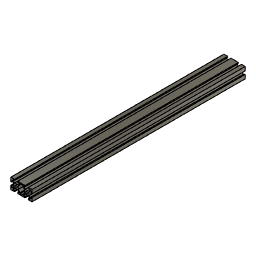
20x40 Extrusion v1 (Autodesk Fusion 360 design; units mm, degrees)
Autodesk Fusion 360 part; units mm, degrees
sketch "Sketch1" plane through (0, 0, 0) normal (0, 1, 0) x (1, 0, 0)
  line L0 (-13, -4) -> (-7, -4)
  line L1 (7, -4) -> (13, -4)
  line L2 (14, -3) -> (14, 3)
  line L3 (13, 4) -> (7, 4)
  line L4 (-7, 4) -> (-13, 4)
  line L5 (-14, 3) -> (-14, -3)
  line L6 (-13, -10) -> (-13, -8)
  line L7 (-7, -10) -> (-7, -8)
  line L8 (7, -10) -> (7, -8)
  line L9 (13, -10) -> (13, -8)
  line L10 (18, -3) -> (20, -3)
  line L11 (18, 3) -> (20, 3)
  line L12 (13, 8) -> (13, 10)
  line L13 (7, 8) -> (7, 10)
  line L14 (-7, 8) -> (-7, 10)
  line L15 (-13, 8) -> (-13, 10)
  line L16 (-18, -3) -> (-20, -3)
  line L17 (-20, 3) -> (-18, 3)
  line L18 (-2.5, -6.3787) -> (-2.5, -8)
  line L19 (2.5, -8) -> (2.5, -6.3787)
  line L20 (2.5, -6.3787) -> (6, -2.8787)
  line L21 (6, -2.8787) -> (6, 2.8787)
  line L22 (6, 2.8787) -> (2.5, 6.3787)
  line L23 (2.5, 6.3787) -> (2.5, 8)
  line L24 (-2.5, 8) -> (-2.5, 6.3787)
  line L25 (-2.5, 6.3787) -> (-6, 2.8787)
  line L26 (-6, 2.8787) -> (-6, -2.8787)
  line L27 (-6, -2.8787) -> (-2.5, -6.3787)
  circle A0 centre (-10, 0) radius 2
  circle A1 centre (10, 0) radius 2
  line L28 (4, -8) -> (4, -7)
  line L29 (4, -7) -> (7, -4)
  line L30 (16, -8) -> (16, -7)
  line L31 (16, -7) -> (13, -4)
  line L32 (18, -6) -> (17, -6)
  line L33 (17, -6) -> (14, -3)
  line L34 (18, 6) -> (17, 6)
  line L35 (17, 6) -> (14, 3)
  line L36 (16, 8) -> (16, 7)
  line L37 (16, 7) -> (13, 4)
  line L38 (7, 4) -> (4, 7)
  line L39 (4, 7) -> (4, 8)
  line L40 (-7, 4) -> (-4, 7)
  line L41 (-4, 7) -> (-4, 8)
  line L42 (-13, 4) -> (-16, 7)
  line L43 (-16, 7) -> (-16, 8)
  line L44 (-18, 6) -> (-17, 6)
  line L45 (-17, 6) -> (-14, 3)
  line L46 (-14, -3) -> (-17, -6)
  line L47 (-17, -6) -> (-18, -6)
  line L48 (-16, -7) -> (-13, -4)
  line L49 (-4, -8) -> (-4, -7)
  line L50 (-4, -7) -> (-7, -4)
  line L51 (-16, -7) -> (-16, -8)
  line L52 (-13, 8) -> (-16, 8)
  line L53 (-13, 10) -> (-20, 10)
  line L54 (16, 8) -> (13, 8)
  line L55 (20, 10) -> (13, 10)
  line L56 (7, 10) -> (-7, 10)
  line L57 (18, -6) -> (18, -3)
  line L58 (18, 3) -> (18, 6)
  line L59 (20, -10) -> (20, -3)
  line L60 (20, 3) -> (20, 10)
  line L61 (13, -8) -> (16, -8)
  line L62 (13, -10) -> (20, -10)
  line L63 (-16, -8) -> (-13, -8)
  line L64 (-20, -10) -> (-13, -10)
  line L65 (-7, -10) -> (7, -10)
  line L66 (-18, 6) -> (-18, 3)
  line L67 (-18, -3) -> (-18, -6)
  line L68 (-20, 10) -> (-20, 3)
  line L69 (-20, -3) -> (-20, -10)
  line L70 (-4, 8) -> (-7, 8)
  line L71 (7, 8) -> (4, 8)
  line L72 (2.5, 8) -> (-2.5, 8)
  line L73 (4, -8) -> (7, -8)
  line L74 (-7, -8) -> (-4, -8)
  line L75 (-2.5, -8) -> (2.5, -8)
  dimension "d4" = 40
  dimension "d5" = 20
  dimension "d7" = 20
  dimension "d8" = 10
  dimension "d9" = 6
  dimension "d10" = 6
  dimension "d11" = 6
  dimension "d12" = 6
  dimension "d13" = 6
  dimension "d14" = 6
  dimension "d15" = 6
  dimension "d16" = 6
  dimension "d17" = 6
  dimension "d18" = 6
  dimension "d19" = 6
  dimension "d20" = 6
  dimension "d21" = 7
  dimension "d22" = 7
  dimension "d23" = 7
  dimension "d24" = 4
  dimension "d25" = 4
  dimension "d26" = 10
  dimension "d27" = 10
  dimension "d28" = 10
  dimension "d29" = 10
  dimension "d30" = 12
  dimension "d32" = 12
  dimension "d33" = 135
  dimension "d34" = 135
  dimension "d35" = 3
  dimension "d36" = 135
  dimension "d37" = 135
  dimension "d38" = 3
  dimension "d39" = 7
  dimension "d41" = 12
  dimension "d42" = 3
  dimension "d43" = 7
  dimension "d44" = 3
  dimension "d45" = 3
  dimension "d46" = 135
  dimension "d47" = 135
  dimension "d48" = 7
  dimension "d49" = 3
  dimension "d50" = 3
  dimension "d52" = 135
  dimension "d53" = 135
  dimension "d54" = 135
  dimension "d55" = 135
  dimension "d56" = 8
  dimension "d57" = 8
  dimension "d58" = 3
  dimension "d59" = 3
  dimension "d60" = 6
  dimension "d61" = 6
  dimension "d62" = 6
  dimension "d63" = 135
  dimension "d64" = 6
  dimension "d65" = 6
  dimension "d66" = 6
  dimension "d67" = 7
  dimension "d68" = 7
  dimension "d69" = 7
  dimension "d70" = 7
  dimension "d71" = 135
  dimension "d72" = 7
  dimension "d73" = 7
  dimension "d74" = 1.5
  dimension "d75" = 1.5
  dimension "d76" = 1.5
  dimension "d77" = 1.5
  dimension "d78" = 1.5
  dimension "d79" = 1.5
  dimension "d80" = 1.5
  dimension "d81" = 1.5
  dimension "d82" = 8
  dimension "d83" = 18
  dimension "d84" = 8
  dimension "d85" = 18
  constraint horizontal L55
  constraint perpendicular L55 L68
  constraint parallel L55 L64
  constraint parallel L59 L68
  constraint perpendicular L0 L57
  constraint parallel L1 L63
  constraint parallel L2 L57
  constraint parallel L3 L54
  constraint parallel L4 L54
  constraint perpendicular L4 L5
  constraint perpendicular L6 L63
  constraint coincident L7.start L64
  constraint coincident L7.end L63
  constraint perpendicular L7 L63
  constraint perpendicular L8 L63
  constraint coincident L9.start L64
  constraint coincident L9.end L63
  constraint perpendicular L9 L63
  constraint perpendicular L10 L59
  constraint coincident L11.start L57
  constraint coincident L11.end L59
  constraint perpendicular L11 L59
  constraint perpendicular L12 L54
  constraint coincident L13.start L54
  constraint coincident L13.end L55
  constraint perpendicular L13 L55
  constraint perpendicular L14 L55
  constraint coincident L15.start L54
  constraint coincident L15.end L55
  constraint perpendicular L15 L54
  constraint coincident L16.start L66
  constraint coincident L16.end L68
  constraint perpendicular L16 L68
  constraint perpendicular L17 L66
  constraint coincident L18.end L63
  constraint perpendicular L18 L63
  constraint coincident L19.start L63
  constraint perpendicular L19 L63
  constraint perpendicular L21 L63
  constraint coincident L23.end L54
  constraint perpendicular L23 L54
  constraint coincident L24.start L54
  constraint perpendicular L24 L54
  constraint perpendicular L26 L54
  constraint coincident L28.start L63
  constraint perpendicular L28 L63
  constraint coincident L30.start L63
  constraint perpendicular L30 L63
  constraint perpendicular L32 L57
  constraint coincident L34.start L57
  constraint perpendicular L34 L57
  constraint perpendicular L36 L54
  constraint perpendicular L3 L39
  constraint coincident L39.end L54
  constraint coincident L41.end L54
  constraint perpendicular L41 L54
  constraint perpendicular L4 L43
  constraint coincident L43.end L54
  constraint perpendicular L44 L66
  constraint coincident L47.end L66
  constraint perpendicular L47 L66
  constraint coincident L49.start L63
  constraint perpendicular L49 L63
  constraint perpendicular L51 L63
  constraint parallel L27 L50
  constraint parallel L20 L29
  constraint parallel L22 L38
  constraint parallel L25 L40
  constraint parallel L54 L55
  constraint parallel L66 L68
  constraint parallel L63 L64
  constraint parallel L57 L59
  constraint collinear L52 L54
  constraint collinear L53 L55
  constraint collinear L54 L71
  constraint collinear L55 L56
  constraint collinear L57 L58
  constraint collinear L59 L60
  constraint collinear L61 L63
  constraint collinear L62 L64
  constraint collinear L63 L74
  constraint collinear L64 L65
  constraint collinear L66 L67
  constraint collinear L68 L69
  constraint collinear L70 L71
  constraint collinear L71 L72
  constraint collinear L73 L74
  constraint collinear L74 L75
  measures "d4" distance of L64.start L59.start
  measures "d5" distance of L53.end L64.start
  measures "d7" distance of origin L59
  measures "d8" distance of origin L55
  measures "d9" distance of L1 L64
  measures "d10" distance of L2 L59
  measures "d11" distance of L3 L55
  measures "d12" distance of L4 L55
  measures "d13" distance of L5 L68
  measures "d14" distance of L0 L64
  measures "d15" distance of L6 L7
  measures "d16" distance of L8 L9
  measures "d17" distance of L10 L11
  measures "d18" distance of L12 L13
  measures "d19" distance of L14 L15
  measures "d20" distance of L16 L17
  measures "d21" distance of L16 L64
  measures "d22" distance of L6 L68
  measures "d23" distance of L9 L59
  measures "d24" diameter of A0
  measures "d25" diameter of A1
  measures "d26" distance of origin A1.centre
  measures "d27" distance of A1.centre L64
  measures "d28" distance of origin A0.centre
  measures "d29" distance of A0.centre L64
  measures "d30" distance of L49 L51
  measures "d32" distance of L28 L30
  measures "d33" angle of L1 L31
  measures "d34" angle of L1 L29
  measures "d35" distance of L6 L51
  measures "d36" angle of L0 L48
  measures "d37" angle of L0 L50
  measures "d38" distance of L8 L28
  measures "d39" distance of L10 L64
  measures "d41" distance of L32 L34
  measures "d42" distance of L10 L32
  measures "d43" distance of L12 L59
  measures "d44" distance of L12 L36
  measures "d45" distance of L13 L39
  measures "d46" angle of L3 L37
  measures "d47" angle of L3 L38
  measures "d48" distance of L15 L68
  measures "d49" distance of L15 L43
  measures "d50" distance of L14 L41
  measures "d52" angle of L4 L42
  measures "d53" angle of L4 L40
  measures "d54" angle of L5 L45
  measures "d55" angle of L5 L46
  measures "d56" distance of L5 L26
  measures "d57" distance of L2 L21
  measures "d58" distance of L16 L47
  measures "d59" distance of L17 L44
  measures "d60" distance of L0.start L0.end
  measures "d61" distance of L1.start L1.end
  measures "d62" distance of L2.start L2.end
  measures "d63" angle of L2 L33
  measures "d64" distance of L3.start L3.end
  measures "d65" distance of L4.start L4.end
  measures "d66" distance of L5.start L5.end
  measures "d67" distance of L5.start L55
  measures "d68" distance of L4.end L68
  measures "d69" distance of L3.start L59
  measures "d70" distance of L2.end L55
  measures "d71" angle of L2 L35
  measures "d72" distance of L1.end L59
  measures "d73" distance of L0.start L68
  measures "d74" distance of L20 L29
  measures "d75" distance of L22 L38
  measures "d76" distance of L25 L40
  measures "d77" distance of L27 L50
  measures "d78" distance of L18 L49
  measures "d79" distance of L19 L28
  measures "d80" distance of L23 L39
  measures "d81" distance of L24 L41
  measures "d82" distance of origin L63
  measures "d83" distance of origin L67
  measures "d84" distance of origin L72
  measures "d85" distance of origin L58
extrude "Extrude1" add sketch "Sketch1" along normal blind 400
